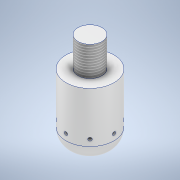
# Autodesk Inventor part: Pintle tip
Saved by Autodesk Inventor 2021 (Build 250183000, 183)
## iProperties
Created: 2022-07-06
Part Number: Pintle tip
Material: Aluminum 6061
Document SubType Name: Modeling
Designer: pc
Density: 2.7 g/cm^3
Appearance: Aluminum - Flat
Mass: 82.3754 g
Surface Area: 63.9622 cm^2
Volume: 30.5094 cm^3
Author: pc
Autodesk Inventor part; units mm, degrees
sketch "Sketch1" plane through (0, 0, 0) normal (0, 1, 0) x (-1, 0, 0)
  circle A0 centre (0, 0) radius 15
  dimension "d0" = 30
  constraints: 1 centre point, 1 coincident
  measures "d0" diameter of A0
extrude "Extrusion1" add sketch "Sketch1" along normal blind 45
sketch "Sketch2" plane through (0, 0, 0) normal (1, 0, 0) x (0, 1, 0)
  point P0 (0, 0)
sketch "Sketch3" plane through (0, 0, 0) normal (1, 0, 0) x (0, 1, 0)
  point P0 (0, 0)
ref_plane "Work Plane1" through (15, 0, 0) normal (1, 0, 0) x (0, 1, 0)
fillet "Fillet2" radius 10 1 edges at (15, 0, 0)
ref_plane "Work Plane2" through (15, 0, 0) normal (1, 0, 0) x (0, 1, 0)
ref_plane "Work Plane3" through (0, 0, 15) normal (0, 0, 1) x (1, 0, 0)
sketch "Sketch8" plane through (0, 0, 15) normal (0, 0, 1) x (1, 0, 0)
  circle A0 centre (0, 14) radius 1
  line L0 (15, 45) -> (-15, 45) projected
  point P0 (0, 0)
  dimension "d19" = 2
  dimension "d20" = 31
  constraints: 1 centre point
  measures "d19" diameter of A0
  measures "d20" distance from line of A0.centre L0
hole "Hole1" at (0, 14, 15) direction (0, 0, -1) diameter 2 depth 15 tip angle 118
pattern_circular "Circular Pattern1" count 8 over 360 about axis through (0, -10, 0) along (0, 1, 0) of "Hole1"
sketch "Sketch19" plane through (0, 45, 0) normal (0, 1, 0) x (1, 0, 0)
  circle A0 centre (0, 0) radius 15
  dimension "d75" = 30
  constraints: 1 centre point, 1 coincident
  measures "d75" diameter of A0
extrude "Extrusion12" cut sketch "Sketch19" against normal blind 3.541
sketch "Sketch20" plane through (0, 41.459, 0) normal (0, 1, 0) x (1, 0, 0)
  line L0 (0, 0) -> (2.4142, -1) projected
  circle A0 centre (0, 0) radius 7.5
  dimension "d78" = 15
  constraints: 1 centre point, 1 coincident
  measures "d78" diameter of A0
extrude "Extrusion13" add sketch "Sketch20" along normal blind 18.541
thread "Thread8" size "M15x1.5" class "6g" standard "ANSI Metric M Profile" full length
body "Solid1"
